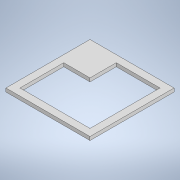
# Autodesk Inventor part: single_meas
Saved by Autodesk Inventor 2020.2 (Build 242310000, 310)
## iProperties
Created: 2021-04-11
Part Number: single_meas
Material: Generic
Document SubType Name: Modeling
Designer: Tarsoly
Density: 1 g/cm^3
Appearance: Default
Author: Tarsoly
Autodesk Inventor part; units mm, degrees
ref_plane "YZ Plane" through (0, 0, 0) normal (1, 0, 0) x (0, 1, 0)
ref_plane "XZ Plane" through (0, 0, 0) normal (0, 1, 0) x (-1, 0, 0)
ref_plane "XY Plane" through (0, 0, 0) normal (0, 0, 1) x (1, 0, 0)
sketch "Sketch1" plane through (0, 0, 0) normal (0, 1, 0) x (-1, 0, 0)
  line L0 (1200, 1200) -> (-1200, 1200)
  line L1 (-1200, 1200) -> (-1200, -1200)
  line L2 (-1200, -1200) -> (1200, -1200)
  line L3 (1200, -1200) -> (1200, 1200)
  line L4 (1200, 1200) -> (-1200, -1200) construction
  line L5 (-1200, 1200) -> (1200, -1200) construction
  line L6 (1000, 1000) -> (1000, -250)
  line L7 (1000, 1000) -> (2250, 1000) construction
  line L8 (1000, -250) -> (250, -250)
  line L9 (250, -250) -> (250, -1000)
  line L10 (250, -1000) -> (-1000, -1000)
  line L11 (-1000, -1000) -> (-1000, 1000)
  line L12 (-1000, 1000) -> (1000, 1000)
  point P0 (0, 0)
  dimension "d0" = 2400
  dimension "d1" = 2400
  dimension "d2" = 1250
  dimension "d3" = 90
  dimension "d4" = 750
  dimension "d5" = 750
  dimension "d6" = 1250
  dimension "d7" = 2000
  constraints: 26 end point, 4 perpendicular, 3 horizontal, 3 point on line, 2 midpoint, 2 parallel, 1 vertical
  measures "d0" distance of L2.end L1.end
  measures "d1" distance of L1.end L0.end
  measures "d2" distance of L6.start L6.end
  measures "d3" angle of L6 L7
  measures "d4" distance of L6.end L8.end
  measures "d5" distance of L8.end L9.end
  measures "d6" distance of L9.end L10.end
  measures "d7" distance of L10.end L11.end
extrude "Extrusion1" add sketch "Sketch1" along normal blind 100
body "Solid1"
